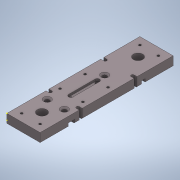
# Autodesk Inventor part: RD53A-2x2_hdi_pickup_tool_v2
Saved by Autodesk Inventor 2021 (Build 250183000, 183)
## iProperties
Created: 2020-12-02
Part Number: RD53A-2x2_hdi_pickup_tool_v2
Material: Aluminum 6061
Document SubType Name: Modeling
Designer: mjones
Density: 2.7 g/cm^3
Appearance: Aluminum Cast
Author: mjones
Autodesk Inventor part; units mm, degrees
ref_plane "YZ Plane" through (0, 0, 0) normal (1, 0, 0) x (0, 1, 0)
ref_plane "XZ Plane" through (0, 0, 0) normal (0, 1, 0) x (-1, 0, 0)
ref_plane "XY Plane" through (0, 0, 0) normal (0, 0, 1) x (1, 0, 0)
sketch "Sketch1" plane through (0, 0, 0) normal (0, 0, 1) x (1, 0, 0)
  line L0 (0, 0) -> (22.5, 0)
  line L1 (22.5, 0) -> (22.5, 90)
  line L2 (22.5, 90) -> (0, 90)
  line L3 (0, 90) -> (0, 0)
  dimension "d0" = 22.5
  dimension "d1" = 90
  constraints: 8 end point, 2 parallel, 1 horizontal, 1 perpendicular
  measures "d0" distance between parallel lines of L1 L3
  measures "d1" distance between parallel lines of L0 L2
extrude "Extrusion1" add sketch "Sketch1" along normal blind 6.35
sketch "Sketch2" plane through (0, 0, 0) normal (0, 0, -1) x (-1, 0, 0)
  line L0 (0, 0) -> (-22.5, 0) projected
  line L1 (-22.5, 90) -> (0, 90) projected
  line L2 (-11.25, 80) -> (-11.25, 10) construction
  line L3 (0, 71) -> (0, 68.55)
  line L4 (-22.5, 68.55) -> (-22.5, 71)
  line L5 (0, 0) -> (-22.5, 0) projected
  line L6 (0, 19) -> (0, 23.45)
  line L7 (-2.5, 23.45) -> (-2.5, 68.55)
  line L8 (-20, 23.45) -> (-20, 68.55)
  line L9 (0, 23.45) -> (-2.5, 23.45)
  line L10 (-20, 23.45) -> (-22.5, 23.45)
  line L11 (-20, 68.55) -> (-22.5, 68.55)
  line L12 (-22.5, 23.45) -> (-22.5, 19)
  line L13 (-2.5, 68.55) -> (0, 68.55)
  line L14 (0, 19) -> (-22.5, 19)
  line L15 (0, 71) -> (-22.5, 71)
  point P0 (0, 71)
  point P1 (-22.5, 19)
  point P2 (0, 19)
  dimension "d7" = 90
  dimension "d9" = 70
  dimension "d10" = 10
  dimension "d85" = 45.1
  dimension "d123" = 45.1
  dimension "d124" = 23.45
  dimension "d126" = 2.5
  dimension "d127" = 2.5
  dimension "d130" = 22.5
  dimension "d151" = 19
  dimension "d152" = 19
  constraints: 26 end point, 2 perpendicular, 1 collinear, 1 parallel, 1 vertical
  measures "d7" distance between parallel lines of L1 L0
  measures "d9" distance of L2.start L2.end
  measures "d10" distance from line of L0 L2.end
  measures "d85" distance between parallel lines of L10 L11
  measures "d123" distance of L7.end L7.start
  measures "d124" distance between parallel lines of L0 L9
  measures "d126" distance between parallel lines of L12 L8
  measures "d127" distance between parallel lines of L6 L7
  measures "d130" distance between parallel lines of L3 L4
  measures "d151" distance between parallel lines of L0 L14
  measures "d152" distance between parallel lines of L1 L15
extrude "Extrusion2" cut sketch "Sketch2" against normal blind 2.5
chamfer "Chamfer1" distance 0.5 angle 45 10 edges at (0, 46, 0) (0, 9.5, 0) (0, 80.5, 0) (22.5, 46, 0) (22.5, 80.5, 0) (22.5, 9.5, 0) (11.25, 0, 0) (11.25, 19, 0) (11.25, 71, 0) (11.25, 90, 0)
sketch "Sketch3" plane through (0, 0, 2.5) normal (0, 0, -1) x (-1, 0, 0)
  line L0 (-15.9, 65) -> (-6.6, 65)
  line L1 (-6.6, 65) -> (-6.6, 66.5)
  line L2 (-6.6, 66.5) -> (-15.9, 66.5)
  line L3 (-15.9, 66.5) -> (-15.9, 65)
  line L4 (-11.25, 17.221) -> (-11.25, 80.5776) construction
  circle A0 centre (-11.25, 49.95) radius 3.5
  circle A1 centre (-11.25, 30.45) radius 5
  line L5 (-0.5, 68.55) -> (-2.5, 68.55) projected
  line L6 (0, 90) -> (-22.5, 90) projected
  point P0 (-11.25, 25.45)
  point P1 (-11.25, 35.45)
  point P2 (-11.25, 53.45)
  point P3 (-11.25, 46.45)
  dimension "d32" = 1.5
  dimension "d120" = 7
  dimension "d121" = 10
  dimension "d174" = 23.5
  constraints: 10 end point, 4 point on circle, 2 centre point, 2 parallel, 2 point on line, 1 horizontal, 1 perpendicular, 1 vertical
  measures "d32" distance between parallel lines of L2 L0
  measures "d120" diameter of A0
  measures "d121" diameter of A1
  measures "d174" distance between parallel lines of L6 L2
extrude "Extrusion3" add sketch "Sketch3" along normal blind 2.5
sketch "Sketch4" plane through (0, 0, 6.35) normal (0, 0, 1) x (1, 0, 0)
  line L0 (11.25, 85.0442) -> (11.25, -17.6533) construction
  line L1 (0, 90) -> (0, 0) construction
  line L2 (22.5, 0) -> (22.5, 90) construction
  line L3 (0, 0) -> (22.5, 0) construction
  line L4 (22.5, 90) -> (0, 90) construction
  point P0 (11.25, 77.5)
  point P1 (11.25, 12.5)
  dimension "d38" = 22.5
  dimension "d39" = 90
  dimension "d40" = 11.25
  dimension "d41" = 65
  dimension "d42" = 12.5
  constraints: 2 end point, 2 point on line, 1 vertical
  measures "d38" distance between parallel lines of L1 L2
  measures "d39" distance between parallel lines of L3 L4
  measures "d40" distance between parallel lines of L1 L0
  measures "d41" distance of point (11.25, 12.5) point (11.25, 77.5)
  measures "d42" distance from line of L4 point (11.25, 77.5)
hole "Hole1" at (11.25, 77.5, 6.35) at (11.25, 12.5, 6.35) direction (0, 0, -1) diameter 6.35 end through all
sketch "Sketch5" plane through (0, 0, 0) normal (0, 0, -1) x (-1, 0, 0)
  line L0 (-11.25, -8.0361) -> (-11.25, 87.9177) construction
  line L1 (-22.5, 0) -> (0, 0) projected
  point P0 (-11.25, 32)
  point P1 (-11.25, 49.95)
  dimension "d153" = 32
  dimension "d154" = 49.95
  constraints: 2 end point, 2 point on line, 1 vertical
  measures "d153" distance from line of L1 point (-11.25, 32)
  measures "d154" vertical distance of L1.end point (-11.25, 49.95)
hole "Hole2" at (11.25, 32, 0) at (11.25, 49.95, 0) direction (0, 0, 1) diameter 2.5 end through all
chamfer "Chamfer3" distance 0.5 angle 45 2 edges at (11.25, 30.75, 0) (11.25, 48.7, 0)
sketch "Sketch6" plane through (0, 0, 6.35) normal (0, 0, 1) x (1, 0, 0)
  line L0 (3.5, -4.6232) -> (3.5, 89.7157) construction
  line L1 (19, -4.6232) -> (19, 89.7157) construction
  line L2 (0, 90) -> (0, 0) construction
  line L3 (22.5, 0) -> (22.5, 90) construction
  line L4 (-5.0643, 32.45) -> (29.6978, 32.45) construction
  line L5 (-5.0643, 49.45) -> (37.041, 49.45) construction
  point P0 (22.5, 68.55)
  point P1 (22.5, 23.45)
  point P2 (3.5, 32.45)
  point P3 (3.5, 49.45)
  point P4 (19, 49.45)
  point P5 (19, 32.45)
  dimension "d69" = 3.5
  dimension "d70" = 3.5
  dimension "d72" = 9
  dimension "d87" = 17
  constraints: 8 end point, 8 point on line, 2 horizontal, 2 vertical
  measures "d69" distance between parallel lines of L0 L2
  measures "d70" distance between parallel lines of L3 L1
  measures "d72" distance from line of L4 point (22.5, 23.45)
  measures "d87" distance between parallel lines of L5 L4
hole "Hole3" at (3.5, 32.45, 6.35) at (3.5, 49.45, 6.35) at (19, 49.45, 6.35) at (19, 32.45, 6.35) direction (0, 0, -1) diameter 1.567 end through all thread size "M2x0.4" class "6H" standard "ANSI Metric M Profile"
sketch "Sketch7" plane through (0, 0, 6.35) normal (0, 0, 1) x (1, 0, 0)
  circle A0 centre (11.25, 49.95) radius 1.25 projected
  arc A1 (12.75, 49.95) -> (9.75, 49.95) centre (11.25, 49.95) ccw
  circle A2 centre (11.25, 32) radius 1.25 projected
  arc A3 (9.75, 32) -> (12.75, 32) centre (11.25, 32) ccw
  line L0 (12.75, 49.95) -> (12.75, 32)
  line L1 (9.75, 49.95) -> (9.75, 32)
  point P0 (0, 0)
  dimension "d155" = 3
  constraints: 4 end point, 4 point on circle, 4 tangent, 2 centre point, 2 coincident, 1 parallel
  measures "d155" distance between parallel lines of L0 L1
extrude "Extrusion4" cut sketch "Sketch7" against normal blind 1.5
sketch "Sketch8" plane through (0, 0, 2.5) normal (0, 0, -1) x (-1, 0, 0)
  line L0 (-22.5, 68.55) -> (-22.5, 23.45) projected
  line L1 (-0.5, 68.55) -> (-2.5, 68.55) projected
  line L2 (-22.5, 0) -> (0, 0) projected
  point P0 (-10.61, 55.55)
  point P1 (-22.5, 90)
  point P2 (-2, 68.55)
  dimension "d89" = 11.89
  dimension "d156" = 55.55
  measures "d89" distance from line of L0 point (-10.61, 55.55)
  measures "d156" distance from line of L2 point (-10.61, 55.55)
hole "Hole4" at (10.61, 55.55, 2.5) direction (0, 0, 1) diameter 3 end through all
chamfer "Chamfer5" distance 1 angle 45 1 edges at (10.61, 54.05, 6.35)
sketch "Sketch9" plane through (0, 0, 6.35) normal (0, 0, 1) x (1, 0, 0)
  point P0 (0, 0)
sketch "Sketch10" plane through (0, 0, 2.5) normal (0, 0, -1) x (-1, 0, 0)
  line L0 (-27.9511, 21.88) -> (7.7068, 21.88) construction
  line L1 (-2.5, 23.45) -> (0, 23.45) construction
  line L2 (0, 71) -> (0, 0) construction
  line L3 (-22.5, 19) -> (-22.5, 23.45) construction
  line L4 (0, 0) -> (-22.5, 0) projected
  point P0 (-17.05, 21.88)
  point P1 (-5.45, 21.88)
  dimension "d102" = 11.6
  dimension "d148" = 21.88
  dimension "d149" = 5.45
  dimension "d150" = 22.5
  constraints: 2 end point, 2 point on line, 1 horizontal
  measures "d102" distance of point (-5.45, 21.88) point (-17.05, 21.88)
  measures "d148" distance from line of L4 point (-5.45, 21.88)
  measures "d149" distance from line of L3 point (-17.05, 21.88)
  measures "d150" distance between parallel lines of L2 L3
hole "Hole5" at (17.05, 21.88, 2.5) at (5.45, 21.88, 2.5) direction (0, 0, 1) diameter 3 end through all
chamfer "Chamfer6" distance 1 angle 45 2 edges at (5.45, 20.38, 6.35) (17.05, 20.38, 6.35)
chamfer "Chamfer7" distance 0.5 angle 45 2 edges at (16.25, 30.45, 0) (14.75, 49.95, 0)
sketch "Sketch11" plane through (0, 0, 6.35) normal (0, 0, 1) x (1, 0, 0)
  line L0 (0, 26.45) -> (2, 26.45)
  line L1 (2, 28.45) -> (0, 28.45)
  line L2 (0, 28.45) -> (0, 26.45)
  arc A0 (2, 26.45) -> (2, 28.45) centre (2, 27.45) ccw
  line L3 (0, 0) -> (22.5, 0) projected
  line L4 (0, 90) -> (0, 0) projected
  line L5 (11.25, 9.2186) -> (11.25, 64.5253) construction
  line L6 (0, 63.55) -> (2, 63.55)
  line L7 (2, 65.55) -> (0, 65.55)
  line L8 (0, 65.55) -> (0, 63.55)
  arc A1 (2, 63.55) -> (2, 65.55) centre (2, 64.55) ccw
  line L9 (22.5, 26.45) -> (20.5, 26.45)
  line L10 (20.5, 28.45) -> (22.5, 28.45)
  line L11 (22.5, 28.45) -> (22.5, 26.45)
  arc A2 (20.5, 28.45) -> (20.5, 26.45) centre (20.5, 27.45) ccw
  line L12 (22.5, 63.55) -> (20.5, 63.55)
  line L13 (20.5, 65.55) -> (22.5, 65.55)
  line L14 (22.5, 65.55) -> (22.5, 63.55)
  arc A3 (20.5, 65.55) -> (20.5, 63.55) centre (20.5, 64.55) ccw
  point P0 (0, 65.55)
  dimension "d141" = 2
  dimension "d142" = 26.45
  dimension "d143" = 2
  dimension "d144" = 2
  dimension "d145" = 39.1
  constraints: 26 end point, 10 symmetric about line, 8 point on circle, 4 centre point, 4 tangent, 2 horizontal, 2 parallel, 1 collinear, 1 vertical, 2 other
  measures "d141" distance between parallel lines of L1 L0
  measures "d142" distance between parallel lines of L3 L0
  measures "d143" distance from line of L4 A0.centre
  measures "d144" distance between parallel lines of L7 L6
  measures "d145" distance between parallel lines of L0 L7
extrude "Extrusion5" cut sketch "Sketch11" against normal through all
sketch "Sketch12" plane through (0, 0, 6.35) normal (0, 0, 1) x (1, 0, 0)
  line L0 (5, 5) -> (5, 85) construction
  line L1 (5, 85) -> (17.5, 85) construction
  line L2 (17.5, 85) -> (17.5, 5) construction
  line L3 (17.5, 5) -> (5, 5) construction
  line L4 (0, 0) -> (22.5, 0) construction
  line L5 (0, 26.45) -> (0, 0) construction
  line L6 (22.5, 90) -> (0, 90) construction
  line L7 (22.5, 65.55) -> (22.5, 90) construction
  line L8 (0, 90) -> (0, 65.55) projected
  circle A0 centre (11.25, 77.5) radius 3.175 projected
  circle A1 centre (11.25, 12.5) radius 3.175 projected
  dimension "d157" = 5
  dimension "d158" = 5
  dimension "d159" = 5
  dimension "d160" = 5
  dimension "d168" = 12.5
  dimension "d169" = 80
  dimension "d170" = 22.5
  dimension "d171" = 7.5
  dimension "d172" = 7.5
  constraints: 8 end point, 4 coincident, 3 perpendicular, 1 vertical
  measures "d157" distance between parallel lines of L4 L3
  measures "d158" distance between parallel lines of L5 L0
  measures "d159" distance between parallel lines of L6 L1
  measures "d160" distance between parallel lines of L7 L2
  measures "d168" distance between parallel lines of L2 L0
  measures "d169" distance between parallel lines of L3 L1
  measures "d170" distance between parallel lines of L7 L8
  measures "d171" distance from line of L1 A0.centre
  measures "d172" distance from line of L3 A1.centre
hole "Hole6" at (5, 85, 6.35) at (17.5, 85, 6.35) at (17.5, 5, 6.35) at (5, 5, 6.35) direction (0, 0, -1) diameter 1.567 end through all thread size "M2x0.4" class "6H" standard "ANSI Metric M Profile"
sketch "Sketch13" plane through (0, 0, 2.5) normal (0, 0, -1) x (-1, 0, 0)
  point P0 (0, 0)
equation "\"d10\" = -0.5 * d9 + 0.5 * d7"
equation "\"d85\" = d123"
equation "\"d40\" = 0.5 * d38"
equation "\"d42\" = -0.5 * d41 + 0.5 * d39"
equation "\"d149\" = -0.5 * d102 + 0.5 * d150"
equation "\"d14\" = -0.5 * d13 + 0.5 * d7"
equation "\"d13\" = 41.1"
body "Solid1"
